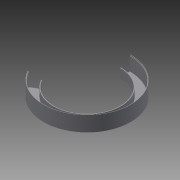
# Autodesk Inventor part: Bottom
Saved by Autodesk Inventor 2015 (Build 190159000, 159)
## iProperties
Created: 2016-03-23
Part Number: Bottom
Material: Generic
Document SubType Name: Modeling
Designer: david_000
Density: 1 g/cm^3
Appearance: Default
Author: david_000
Autodesk Inventor part; units mm, degrees
ref_plane "YZ Plane" through (0, 0, 0) normal (1, 0, 0) x (0, 1, 0)
ref_plane "XZ Plane" through (0, 0, 0) normal (0, 1, 0) x (-1, 0, 0)
ref_plane "XY Plane" through (0, 0, 0) normal (0, 0, 1) x (1, 0, 0)
sketch "Sketch1" plane through (0, 0, 0) normal (1, 0, 0) x (0, 1, 0)
  line L0 (0, 0) -> (-36.83, 0)
  line L1 (-36.83, 0) -> (-36.83, -44.45)
  line L2 (-36.83, -44.45) -> (26.67, -44.45)
  line L3 (26.67, -44.45) -> (26.67, -42.8625)
  line L4 (26.67, -42.8625) -> (23.495, -42.8625)
  line L5 (23.495, -42.8625) -> (23.495, -41.275)
  line L6 (0, 0) -> (0, -3.175)
  line L7 (0, -3.175) -> (-33.655, -3.175)
  line L8 (-33.655, -3.175) -> (-33.655, -41.275)
  line L9 (-33.655, -41.275) -> (22.225, -41.275)
  line L10 (51.7821, 139.7) -> (-41.1614, 139.7)
  line L11 (23.495, -41.275) -> (22.225, -41.275)
  dimension "d10" = 36.83
  dimension "d11" = 44.45
  dimension "d12" = 63.5
  dimension "d13" = 1.5875
  dimension "d14" = 3.175
  dimension "d15" = 1.5875
  dimension "d16" = 3.175
  dimension "d17" = 33.655
  dimension "d18" = 38.1
  dimension "d19" = 139.7
  dimension "d20" = 55.88
  constraints: 24 end point, 7 perpendicular, 2 horizontal, 2 vertical
  measures "d10" distance of L0.start L0.end
  measures "d11" distance of L0.end L1.end
  measures "d12" distance of L1.end L2.end
  measures "d13" distance of L2.end L3.end
  measures "d14" distance of L3.end L4.end
  measures "d15" distance of L4.end L5.end
  measures "d16" distance of L0.start L6.end
  measures "d17" distance of L6.end L7.end
  measures "d18" distance of L7.end L8.end
  measures "d19" distance between parallel lines of L0 L10
  measures "d20" distance of L8.end L9.end
revolve "Revolution1" add sketch "Sketch1" angle 240 about axis through (0, 51.7821, 139.7) along (0, -1, 0)
body "Solid1"
